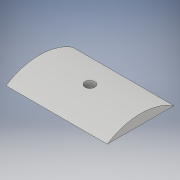
# Autodesk Inventor part: Braket Top V2
Saved by Autodesk Inventor 2019 (Build 230136000, 136)
## iProperties
Created: 2018-11-11
Part Number: Braket Top V2
Material: Generic
Document SubType Name: Modeling
Designer: mrhftc
Density: 1 g/cm^3
Appearance: Default
Author: mrhftc
Autodesk Inventor part; units mm, degrees
ref_plane "YZ Plane" through (0, 0, 0) normal (1, 0, 0) x (0, 1, 0)
ref_plane "XZ Plane" through (0, 0, 0) normal (0, 1, 0) x (-1, 0, 0)
ref_plane "XY Plane" through (0, 0, 0) normal (0, 0, 1) x (1, 0, 0)
sketch "Arc Extrusion" plane through (0, 0, 0) normal (1, 0, 0) x (0, 1, 0)
  line L0 (0, -13.5) -> (0, 13.5)
  arc A0 (0, -13.5) -> (0, 13.5) centre (-20.7812, 0) ccw
  point P0 (0, 0)
  point P1 (4, 0)
  dimension "d5" = 27
  dimension "d6" = 4
  constraints: 3 point on circle, 2 end point, 1 centre point
  measures "d5" distance of L0.start L0.end
  measures "d6" distance of point (0, 0) point (4, 0)
extrude "Main Arc Extrusion" add sketch "Arc Extrusion" along normal blind 41
sketch "Hole Sketch" plane through (0, 0, -13.5) normal (0, -1, 0) x (1, 0, 0)
  circle A0 centre (20.5, 13.5) radius 2
  line L0 (41, 27) -> (41, 0) projected
  line L1 (0, 27) -> (41, 27) projected
  line L2 (0, 0) -> (41, 0) projected
  line L3 (0, 27) -> (0, 0) construction
  point P0 (0, 13.5)
  dimension "d9" = 4
  dimension "d12" = 13.5
  dimension "d13" = 13.5
  dimension "d16" = 20.5
  dimension "d17" = 20.5
  constraints: 1 centre point
  measures "d9" diameter of A0
  measures "d12" distance from line of L1 A0.centre
  measures "d13" distance from line of L2 A0.centre
  measures "d16" distance from line of L0 A0.centre
  measures "d17" distance from line of L3 A0.centre
extrude "Extrusion2" cut sketch "Hole Sketch" against normal through all
body "Solid1"
